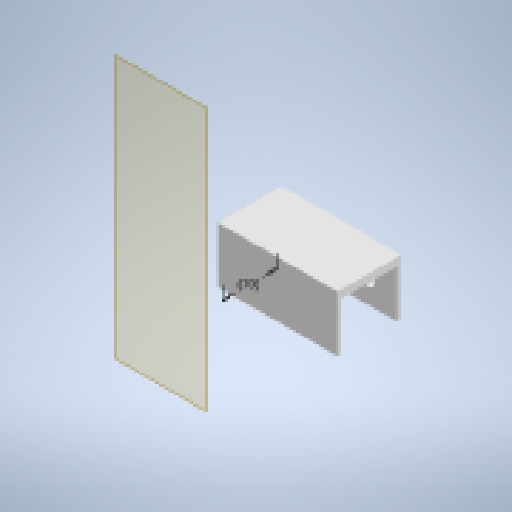
# Autodesk Inventor part: korona
Saved by Autodesk Inventor 2025 (Build 290162000, 162)
## iProperties
Created: 2025-02-05
Part Number: korona
Material: Generic
Document SubType Name: Modeling
Designer: piotr
Density: 1 g/cm^3
Appearance: Default
Author: piotr
Autodesk Inventor part; units mm, degrees
ref_plane "YZ Plane" through (0, 0, 0) normal (1, 0, 0) x (0, 1, 0)
ref_plane "XZ Plane" through (0, 0, 0) normal (0, 1, 0) x (-1, 0, 0)
ref_plane "XY Plane" through (0, 0, 0) normal (0, 0, 1) x (1, 0, 0)
ref_plane "Work Plane1" through (0, 0, 0) normal (0, 0, 1) x (1, 0, 0)
sketch "Sketch1" plane through (0, 0, 0) normal (0, 0, 1) x (1, 0, 0)
  circle A0 centre (114.3836, 12.2466) radius 10 projected
  circle A1 centre (114.3836, 12.2466) radius 10 projected
  line L0 (114.3836, 12.2466) -> (76.8836, 12.2466)
  line L1 (124.7866, -536.2038) -> (-25.2134, -536.2038) projected
  line L2 (114.3836, 12.2466) -> (114.3836, -536.2038)
  line L3 (76.8836, 12.2466) -> (76.8836, 52.1676)
  line L4 (76.8836, 52.1676) -> (226.8836, 52.1676)
  line L5 (226.8836, 52.1676) -> (226.8836, -17.8324)
  line L6 (226.8836, -17.8324) -> (76.8836, -17.8324)
  line L7 (76.8836, -17.8324) -> (76.8836, 12.2466)
  circle A2 centre (114.3836, 12.2466) radius 10 projected
  line L8 (151.8836, 52.1676) -> (151.8836, -17.8324)
  circle A3 centre (189.3836, 12.2466) radius 10
  line L9 (76.8836, 52.1676) -> (76.8836, 42.1676)
  line L10 (76.8836, 42.1676) -> (226.8836, 42.1676)
  line L11 (226.8836, 52.1676) -> (76.8836, 52.1676)
  line L12 (76.8836, 52.1676) -> (76.8836, 42.1676)
  line L13 (76.8836, 42.1676) -> (226.8836, 42.1676)
  line L14 (226.8836, 42.1676) -> (226.8836, 52.1676)
  point P0 (0, 0)
  dimension "d0" = 37.5
  dimension "d1" = 548.4504
  dimension "d2" = 39.921
  dimension "d3" = 150
  dimension "d4" = 70
  dimension "d5" = 10
  dimension "d6" = 150
  constraints: 28 end point, 4 horizontal, 4 perpendicular, 2 midpoint, 2 parallel, 2 point on line, 2 vertical, 1 centre point, 1 symmetric about line, 1 other
  measures "d0" distance of L0.start L0.end
  measures "d1" distance of L0.start L2.end
  measures "d2" distance of L0.end L3.end
  measures "d3" distance of L3.end L4.end
  measures "d4" distance of L4.end L5.end
  measures "d5" distance of L3.end L9.end
  measures "d6" distance of L9.end L10.end
extrude "Extrusion1" add sketch "Sketch1" along normal blind 5 contours A0 L0 L3 L10 L8 L6 L2 | A0 L2 L6 L7 L0 | L3 L4 L8 L10 | L8 L10 L5 L6 | L8 L4 L5 L10
sketch "Sketch3" plane through (0, 0, 0) normal (0, 0, -1) x (-1, 0, 0)
  line L0 (-226.8836, 52.1676) -> (-76.8836, 52.1676) projected
  line L1 (-76.8836, 42.1676) -> (-226.8836, 42.1676) projected
  line L2 (-226.8836, 52.1676) -> (-76.8836, 52.1676)
  line L3 (-76.8836, 52.1676) -> (-76.8836, 42.1676)
  line L4 (-76.8836, 42.1676) -> (-226.8836, 42.1676)
  line L5 (-226.8836, 42.1676) -> (-226.8836, 52.1676)
  point P0 (0, 0)
  constraints: 8 end point, 2 parallel, 1 horizontal, 1 perpendicular
extrude "Extrusion2" add sketch "Sketch3" along normal blind 80
sketch "Sketch4" plane through (0, 0, -80) normal (0, 0, -1) x (-1, 0, 0)
  line L0 (-226.8836, 52.1676) -> (-76.8836, 52.1676) projected
  line L1 (-76.8836, -17.8324) -> (-226.8836, -17.8324) projected
  line L2 (-226.8836, 52.1676) -> (-76.8836, 52.1676)
  line L3 (-76.8836, 52.1676) -> (-76.8836, -17.8324)
  line L4 (-76.8836, -17.8324) -> (-226.8836, -17.8324)
  line L5 (-226.8836, -17.8324) -> (-226.8836, 52.1676)
  point P0 (0, 0)
  point P1 (-76.8836, 52.1676)
  constraints: 8 end point, 2 parallel, 1 horizontal, 1 perpendicular
extrude "Extrusion3" add sketch "Sketch4" along normal blind 5
sketch "Sketch6" plane through (0, 0, -85) normal (0, 0, -1) x (-1, 0, 0)
  line L0 (-98.3957, 24.2628) -> (62.6208, -189.9747) projected
  arc A0 (-98.3957, 24.2628) -> (-130.3715, 0.2304) centre (-114.3836, 12.2466) ccw projected
  line L1 (30.6451, -214.007) -> (-130.3715, 0.2304) projected
  arc A1 (30.6451, -214.007) -> (62.6208, -189.9747) centre (46.6329, -201.9908) ccw projected
  circle A2 centre (46.6329, -201.9908) radius 9.25 projected
  circle A3 centre (-114.3836, 12.2466) radius 10 projected
  circle A4 centre (-189.3836, 12.2466) radius 10 projected
  point P0 (0, 0)
extrude "Extrusion4" cut sketch "Sketch6" against normal blind 10 contours A3 | A4
sketch "Sketch8" plane through (76.8836, 52.1676, 5) normal (0, 1, 0) x (1, 0, 0)
  line L0 (0, 0) -> (0, 90) projected
  line L1 (150, 0) -> (0, 0) projected
  line L2 (150, 90) -> (150, 0) projected
  line L3 (0, 90) -> (150, 90) projected
  point P0 (-76.8836, 5)
extrude "Extrusion6" add sketch "Sketch8" along normal blind 0.079
body "Solid1"
